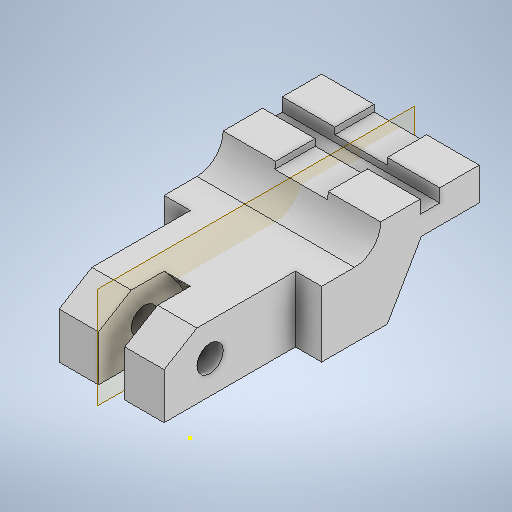
# Autodesk Inventor part: thi1
Saved by Autodesk Inventor 2025.2 (Build 292293000, 293)
## iProperties
Created: 2024-12-05
Part Number: thi1
Material: Generic
Document SubType Name: Modeling
Designer: hongquan
Density: 1 g/cm^3
Appearance: Default
Author: hongquan
Autodesk Inventor part; units mm, degrees
ref_plane "XZ Plane" through (0, 0, 0) normal (0, 1, 0) x (-1, 0, 0)
ref_plane "XY Plane" through (0, 0, 0) normal (0, 0, 1) x (1, 0, 0)
sketch "Sketch1" plane through (0, 0, 0) normal (1, 0, 0) x (0, 1, 0)
  point P0 (0, 0)
sketch "Sketch2" plane through (0, 0, 0) normal (1, 0, 0) x (0, 1, 0)
  line L0 (70, -220) -> (0, -220) construction
  line L1 (0, -220) -> (0, 0) construction
  circle A0 centre (25, -35) radius 10
  line L2 (0, 0) -> (0, -150)
  line L3 (0, -150) -> (161.1976, -150) construction
  line L4 (70, -220) -> (45, -220)
  line L5 (70, -220) -> (70, -145)
  line L6 (70, -145) -> (70, -145)
  line L7 (50, -125) -> (50, 0) construction
  line L8 (50, 0) -> (0, 0) construction
  arc A1 (50, -125) -> (70, -145) centre (70, -125) ccw
  line L9 (50, -25) -> (35, 0)
  line L10 (0, -150) -> (116.4137, -150) construction
  line L11 (45, -220) -> (45, -175.9808)
  line L12 (50, -25) -> (50, -125)
  line L13 (35, 0) -> (0, 0)
  line L14 (0, -150) -> (45, -175.9808)
  line L15 (50, 0) -> (50, -50)
  line L16 (0, 0) -> (0, -75)
  circle A2 centre (-13.259, 14.018) radius 90 construction
  arc A3 (0, -75) -> (50, -50) centre (-13.259, 14.018) ccw
  line L17 (70, -190) -> (70, -175)
  line L18 (70, -175) -> (60, -175)
  line L19 (60, -175) -> (60, -190)
  line L20 (60, -190) -> (70, -190)
  point P0 (35, 0)
  point P1 (50, -145)
  point P2 (17.5, 0)
  dimension "d0" = 220
  dimension "d1" = 70
  dimension "d2" = 20
  dimension "d5" = 25
  dimension "d7" = 150
  dimension "d9" = 25
  dimension "d10" = 75
  dimension "d12" = 20
  dimension "d13" = 20
  dimension "d14" = 25
  dimension "d15" = 15
  dimension "d17" = 35
  dimension "d25" = 50
  dimension "d26" = 75
  dimension "d27" = 180
  dimension "d28" = 30
  dimension "d29" = 15
  dimension "d30" = 10
  constraints: 42 end point, 8 point on line, 6 horizontal, 6 point on circle, 5 vertical, 4 centre point, 3 tangent, 2 midpoint, 2 perpendicular, 1 coincident, 1 other
  measures "d0" distance of L0.end L1.end
  measures "d1" distance of L0.start L0.end
  measures "d2" diameter of A0
  measures "d5" distance from line of L1 A0.centre
  measures "d7" distance of L1.end L2.end
  measures "d9" distance of L0.start L4.end
  measures "d10" distance of L0.start L5.end
  measures "d12" distance of L5.end point (50, -145)
  measures "d13" radius of A1
  measures "d14" distance from line of L8 L9.start
  measures "d15" distance of L7.end L9.end
  measures "d17" vertical distance of point (17.5, 0) A0.centre
  measures "d25" distance of L7.end L15.end
  measures "d26" distance of L1.end L16.end
  measures "d27" diameter of A2
  measures "d28" distance of L17.start L0.start
  measures "d29" distance of L17.start L17.end
  measures "d30" distance of L17.end L18.end
extrude "Extrusion1" add sketch "Sketch2" against normal blind 120
sketch "Sketch3" plane through (0, 70, -145) normal (0, 1, 0) x (1, 0, 0)
  line L0 (0, -145) -> (-120, -145) projected
  line L1 (-60, -145) -> (-60, 75)
  line L2 (0, 75) -> (-120, 75) projected
  line L3 (-120, -145) -> (-120, 75)
  line L4 (-120, 75) -> (0, 75)
  line L5 (0, -145) -> (-120, -145)
  line L6 (0, -145) -> (0, 75)
  line L7 (-100, -145) -> (-20, -145)
  line L8 (-20, -145) -> (-20, -45)
  line L9 (0, 30.9808) -> (-120, 30.9808) projected
  line L10 (-100, -145) -> (-100, -45)
  line L11 (-100, -45) -> (-120, -45)
  line L12 (-20, -45) -> (0, -45)
  dimension "d21" = 80
  dimension "d22" = 100
  constraints: 20 end point, 4 point on line, 3 midpoint, 3 perpendicular, 2 equal length, 1 collinear, 1 horizontal, 1 symmetric about line, 1 vertical
  measures "d21" distance of L7.start L7.end
  measures "d22" distance of L7.end L8.end
extrude "Extrusion2" cut sketch "Sketch3" against normal blind 120 contours L0 L8 L12 L6 | L0 L3 L11 L10
extrude "Extrusion3" cut sketch "Sketch2" against normal blind 120 contours L5 L20 L19 L18
ref_plane "Work Plane1" through (-60, 35, 0) normal (1, 0, 0) x (0, 1, 0)
sketch "Sketch4" plane through (-60, 35, 0) normal (1, 0, 0) x (0, 1, 0)
  line L0 (-35, 0) -> (0, 0) projected
  line L1 (-35, 0) -> (0, 0)
  line L2 (0, 0) -> (15, -25) projected
  line L3 (0, 0) -> (15, -25)
  line L4 (-35, 0) -> (-35, -75)
  arc A0 (-35, -75) -> (15, -50) centre (-48.259, 14.018) ccw
  line L5 (15, 0) -> (15, -50)
  line L6 (15, -25) -> (15, -100) projected
  line L7 (15, -50) -> (15, -100)
  line L8 (15, -100) -> (-35, -100)
  line L9 (-35, -100) -> (-35, -75)
  line L10 (15, 0) -> (-35, 0)
  dimension "d9" = 25
  dimension "d33" = 75
  dimension "d34" = 180
  dimension "d35" = 50
  constraints: 16 end point, 3 perpendicular, 2 collinear, 2 point on circle, 2 vertical, 1 centre point, 1 horizontal, 1 point on line
  measures "d33" distance of L0.start L4.end
  measures "d34" diameter of A0
  measures "d35" distance of L5.start L5.end
extrude "Extrusion4" cut sketch "Sketch4" along normal mid plane 20 contours L0 L2 L5 A0 L4
sketch "Sketch5" plane through (0, 45, -220) normal (0, 0, -1) x (-1, 0, 0)
  line L0 (0, 25) -> (120, 25) projected
  line L1 (60, 25) -> (60, -45) construction
  line L2 (40, 20) -> (80, 20)
  line L3 (40, 20) -> (40, 25)
  line L4 (80, 20) -> (80, 25)
  line L5 (40, 25) -> (80, 25)
  point P0 (0, -45)
  point P1 (60, 20)
  dimension "d38" = 40
  dimension "d39" = 5
  constraints: 10 end point, 3 point on line, 2 midpoint, 2 vertical, 1 collinear, 1 horizontal, 1 perpendicular
  measures "d38" distance of L2.start L2.end
  measures "d39" distance between parallel lines of L0 L2
extrude "Extrusion5" cut sketch "Sketch5" against normal blind 200
body "Solid1"
